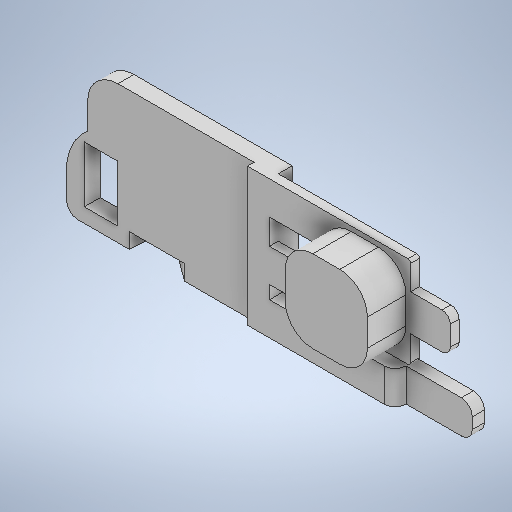
# Autodesk Inventor part: Botão Liga Desliga Monitor LG E2011
Saved by Autodesk Inventor 2025.3 (Build 293356000, 356)
## iProperties
Created: 2025-07-08
Part Number: Botão Liga Desliga Monitor LG E2011
Material: Genérico
Document SubType Name: Modeling
Designer: user
Density: 1 g/cm^3
Appearance: Padrão
Author: user
## iProperties of the stored document Botão Liga Desliga Monitor LG E2011_3DPrint.ipt
Created: 2025-07-08
Part Number: Botão Liga Desliga Monitor LG E2011_3DPrint
Material: Genérico
Document SubType Name: Modeling
Designer: user
Density: 1 g/cm^3
Appearance: Padrão
Author: user
Autodesk Inventor part; units mm, degrees
ref_plane "YZ Plane" through (0, 0, 0) normal (1, 0, 0) x (0, 1, 0)
ref_plane "XZ Plane" through (0, 0, 0) normal (0, 1, 0) x (-1, 0, 0)
ref_plane "XY Plane" through (0, 0, 0) normal (0, 0, 1) x (1, 0, 0)
sketch "Esboço1" plane through (0, 0, 0) normal (0, 0, 1) x (1, 0, 0)
  line L0 (0, 0) -> (36.4, 0)
  line L1 (0, 6.25) -> (36.4, 6.25)
  line L2 (36.4, 6.25) -> (36.4, -6.25)
  line L3 (36.4, -6.25) -> (0, -6.25)
  line L4 (0, -6.25) -> (0, 6.25)
  dimension "d0" = 36.4
  constraints: 10 end point, 2 horizontal, 2 parallel, 1 perpendicular
  measures "d0" distance of L0.start L0.end
extrude "Extrusão1" add sketch "Esboço1" along normal blind 2.65
sketch "Esboço2" plane through (0, 0, 2.65) normal (0, 0, 1) x (1, 0, 0)
  line L0 (0, -6.25) -> (36.4, -6.25) projected
  line L1 (19, -6.25) -> (19, -16.3254)
  line L2 (36.4, 6.25) -> (0, 6.25) projected
  line L3 (19, -6.25) -> (0, -6.25)
  line L4 (0, -6.25) -> (0, 6.25)
  line L5 (0, 6.25) -> (19, 6.25)
  line L6 (19, 6.25) -> (19, -6.25)
  line L7 (36.4, -6.25) -> (36.4, 6.25) projected
  line L8 (17, -6.25) -> (12.9263, -12.0226)
  line L9 (17, -6.25) -> (0, -6.25)
  line L10 (0, -6.25) -> (0, 6.25)
  line L11 (0, 6.25) -> (17, 6.25)
  line L12 (17, 6.25) -> (17, -6.25)
  point P0 (0, 0)
  dimension "d6" = 17.4
  constraints: 20 end point, 4 parallel, 2 horizontal, 2 perpendicular, 2 point on line
  measures "d6" distance between parallel lines of L7 L1
extrude "Extrusão2" cut sketch "Esboço2" against normal blind 0.6 contours L4 L2 L12 L0
sketch "Esboço3" plane through (0, 0, 2.05) normal (0, 0, 1) x (1, 0, 0)
  line L0 (17, 6.25) -> (17, -6.25) projected
  line L1 (17, 6.25) -> (1.9, 6.25)
  line L2 (36.4, 6.25) -> (0, 6.25) projected
  line L3 (1.9, 6.25) -> (1.9, 17.1493)
  line L4 (1.9, 6.25) -> (1.9, 0.15)
  line L5 (0, 6.25) -> (0, -6.25) projected
  line L6 (0, -6.25) -> (36.4, -6.25) projected
  line L7 (0, -4.95) -> (1.6, -4.95)
  line L8 (1.6, -4.95) -> (1.6, 0.15)
  line L9 (1.6, 0.15) -> (1.9, 0.15)
  line L10 (1.6, -4.95) -> (1.6, -7.116)
  line L11 (1.6, -4.95) -> (4.6, -4.95)
  line L12 (4.6, -4.95) -> (4.6, 0.15)
  line L13 (4.6, 0.15) -> (1.6, 0.15)
  line L14 (1.6, 0.15) -> (1.6, -4.95)
  line L15 (0, 0.15) -> (0, -2.35)
  line L16 (1.6, 0.15) -> (1.2464, 0.5036)
  line L17 (1.6, 0.15) -> (2.1, 0.15) construction
  line L18 (1.9, 0.15) -> (1.9, 1.15)
  arc A0 (1.9, 1.15) -> (0, -2.35) centre (5.3437, -2.9852) ccw
  point P0 (0, 0)
  dimension "d11" = 6.1
  dimension "d13" = 1.6
  dimension "d14" = 3
  dimension "d15" = 1.9
  dimension "d16" = 2.5
  dimension "d17" = 0.5
  dimension "d18" = 135
  dimension "d19" = 1
  constraints: 30 end point, 6 point on line, 3 horizontal, 3 perpendicular, 2 parallel, 2 point on circle, 2 vertical, 1 centre point, 1 equal length
  measures "d11" distance of L1.end L4.end
  measures "d13" distance of L7.start L7.end
  measures "d14" distance of L13.end L12.end
  measures "d15" distance between parallel lines of L5 L4
  measures "d16" distance of L15.start L15.end
  measures "d17" distance of L13.end L16.end
  measures "d18" angle of L17 L16
  measures "d19" distance of L4.end L18.end
extrude "Extrusão3" cut sketch "Esboço3" against normal blind 3 contours L4 A0 L5 L2 | L8 L9 L13 L12 L11
fillet "Arredondamento1" radius 2.75 1 edges at (1.9, 6.25, 1.025)
fillet "Arredondamento2" radius 1 1 edges at (0, -6.25, 1.025)
sketch "Esboço4" plane through (36.4, -6.25, 0) normal (0, -1, 0) x (1, 0, 0)
  line L0 (-30.7, 2.05) -> (-30.7, 6.0011)
  line L1 (-36.4, 0) -> (-30.6, 0)
  line L2 (-31.8, 0) -> (-34.8, 0) projected
  line L3 (-30.7, 2.05) -> (-30.6, 0)
  line L4 (-30.6, 0) -> (-27.55, 0)
  line L5 (0, 0) -> (-31.75, 0) projected
  line L6 (-27.55, 0) -> (-27.55, 0.7)
  line L7 (-30.7, 2.05) -> (-25.7, 2.05)
  line L8 (-31.75, 2.05) -> (-19.4, 2.05) projected
  line L9 (-27.55, 0.7) -> (-25.7, 2.05)
  point P0 (-36.4, 2.05)
  dimension "d25" = 5.8
  dimension "d26" = 3.05
  dimension "d27" = 0.7
  dimension "d28" = 5
  constraints: 14 end point, 2 point on line, 1 collinear, 1 vertical
  measures "d25" distance of L1.start L1.end
  measures "d26" distance of L1.end L4.end
  measures "d27" distance of L4.end L6.end
  measures "d28" distance of L0.start L7.end
extrude "Extrusão4" cut sketch "Esboço4" against normal blind 1.4
sketch "Esboço5" plane through (0, 0, 0) normal (0, 0, -1) x (-1, 0, 0)
  line L0 (-17, -6.25) -> (-10.7, -6.25) projected
  line L1 (-17, 1.25) -> (-6.1, 1.25)
  line L2 (-4.6, -4.95) -> (-4.6, 0.15) projected
  line L3 (-4.6, -0.25) -> (-4.6, -6.25)
  line L4 (-17, 6.25) -> (-4.6, 6.25)
  arc A0 (-1.9, 3.5) -> (-4.65, 6.25) centre (-4.65, 3.5) ccw projected
  arc A1 (-4.6, 6.2495) -> (-4.65, 6.25) centre (-4.65, 3.5) ccw
  line L5 (-1.9, 1.15) -> (-1.9, 3.5) projected
  line L6 (-1.9, 3.5) -> (-1.9, 1.15)
  arc A2 (0, -2.35) -> (-1.9, 1.15) centre (-5.3437, -2.9852) ccw projected
  line L7 (0, -2.35) -> (0, -5.25) projected
  line L8 (0, -2.35) -> (0, -5.25)
  line L9 (-1, -6.25) -> (-5.8, -6.25) projected
  line L10 (-1, -6.25) -> (-4.6, -6.25)
  arc A3 (-1, -6.25) -> (0, -5.25) centre (-1, -5.25) ccw projected
  arc A4 (-1, -6.25) -> (0, -5.25) centre (-1, -5.25) ccw
  arc A5 (0, -3.6203) -> (-1.9, 1.15) centre (-5.3437, -2.9852) ccw
  line L11 (-6.1, 1.25) -> (-6.1, -0.25)
  arc A6 (-4.6, -0.25) -> (-6.1, 1.25) centre (-6.1, -0.25) ccw
  line L12 (-17, -6.25) -> (-19, -6.25)
  line L13 (-17, -6.25) -> (-36.4, -6.25) projected
  line L14 (-19, -6.25) -> (-19, 6.25)
  line L15 (-19, 6.25) -> (-17, 6.25)
  line L16 (-17, 1.25) -> (-19, 1.25)
  point P0 (0, 0)
  point P1 (-4.6, -0.25)
  dimension "d31" = 7.5
  dimension "d36" = 2
  constraints: 22 end point, 8 point on circle, 6 point on line, 5 perpendicular, 4 centre point, 4 coincident, 3 collinear, 1 horizontal
  measures "d31" distance of L0.start L1.start
  measures "d36" distance of L0.start L12.end
extrude "Extrusão5" cut sketch "Esboço5" against normal blind 0.6 contours L16 L14 L15 L4 A0 L5 A2 L7 A3 L9 L3 L2 A6 L1
sketch "Esboço6" plane through (0, 0, 2.65) normal (0, 0, 1) x (1, 0, 0)
  line L0 (17, -6.25) -> (36.4, -6.25) projected
  line L1 (36.4, -6.25) -> (18.95, -6.25)
  line L2 (18.95, -6.25) -> (18.95, -3.25)
  line L3 (18.95, -3.25) -> (36.4, -3.25)
  line L4 (36.4, -3.25) -> (36.4, -6.25)
  line L5 (36.4, -3.25) -> (30.4, -3.25)
  line L6 (30.4, -3.25) -> (30.4, -6.25)
  line L7 (30.4, -6.25) -> (36.4, -6.25)
  line L8 (36.4, -6.25) -> (36.4, -3.25)
  point P0 (0, 0)
  dimension "d37" = 17.45
  dimension "d38" = 3
  dimension "d39" = 6
  constraints: 16 end point, 4 parallel, 2 horizontal, 2 perpendicular, 1 point on line
  measures "d37" distance of L2.end L3.end
  measures "d38" distance of L1.end L2.end
  measures "d39" distance of L7.end L6.end
extrude "Extrusão6" cut sketch "Esboço6" against normal blind 1 contours L6 L3 L4 L0
sketch "Esboço7" plane through (0, 0, 0) normal (0, 0, -1) x (-1, 0, 0)
  line L0 (-8.85, -6.25) -> (-36.4, -6.25) projected
  line L1 (-36.4, -6.25) -> (-29.3, -6.25)
  line L2 (-29.3, -6.25) -> (-29.3, -3.25)
  line L3 (-29.3, -3.25) -> (-36.4, -3.25)
  line L4 (-36.4, -3.25) -> (-36.4, -6.25)
  point P0 (0, 0)
  dimension "d42" = 7.1
  constraints: 8 end point, 2 parallel, 1 horizontal, 1 perpendicular
  measures "d42" distance of L3.end L2.end
extrude "Extrusão7" cut sketch "Esboço7" against normal blind 0.55
fillet "Arredondamento3" radius 1 1 edges at (30.4, -4.75, 2.65)
fillet "Arredondamento4" radius 2.5 1 edges at (29.3, -4.75, 0)
sketch "Esboço8" plane through (0, 0, 2.65) normal (0, 0, 1) x (1, 0, 0)
  line L0 (19, 6.25) -> (31.8, 6.25)
  line L1 (31.8, -2.05) -> (19, -2.05)
  line L2 (31.8, 3.775) -> (36.4, 3.775)
  line L3 (36.4, 0.475) -> (31.8, 0.475)
  line L4 (31.8, 6.25) -> (31.8, 3.775)
  line L5 (31.8, 0.475) -> (31.8, -2.05)
  line L6 (31.8, 6.25) -> (31.8, 3.775)
  line L7 (31.8, 0.475) -> (31.8, -2.05)
  line L8 (19, 6.25) -> (19, -2.05)
  line L9 (36.4, -3.25) -> (36.4, 6.25) projected
  line L10 (36.4, -3.25) -> (29.3, -3.25) projected
  line L11 (36.4, -3.25) -> (19, -3.25)
  line L12 (19, -3.25) -> (19, -2.05)
  line L13 (36.4, -3.25) -> (36.4, 0.475)
  line L14 (36.4, 3.775) -> (36.4, 6.25)
  line L15 (36.4, 3.775) -> (36.4, 0.475)
  line L16 (36.4, -3.25) -> (36.4, 6.25) projected
  line L17 (31.8, 3.775) -> (36.4, 3.775)
  line L18 (36.4, 3.775) -> (36.4, 6.25)
  line L19 (36.4, 6.25) -> (31.8, 6.25)
  line L20 (31.8, 6.25) -> (31.8, 3.775)
  point P0 (0, 0)
  dimension "d51" = 8.3
  dimension "d54" = 17.4
  constraints: 36 end point, 4 point on line, 3 horizontal, 3 parallel, 2 collinear, 2 perpendicular, 2 vertical
  measures "d51" distance of L5.end L4.start
  measures "d54" distance between parallel lines of L9 L8
extrude "Extrusão8" cut sketch "Esboço8" against normal blind 3 contours L19 L9 L2 L4 | L1 L5 L3 L9 L10 L11 L12
fillet "Arredondamento5" radius 0.75 2 edges at (36.4, 0.475, 1.325) (36.4, 3.775, 1.325)
fillet "Arredondamento6" radius 1 2 edges at (36.4, -6.25, 1.1) (36.4, -3.25, 1.1)
sketch "Esboço9" plane through (0, 0, 2.65) normal (0, 0, 1) x (1, 0, 0)
  line L0 (19, 6.25) -> (19, 3.25)
  line L1 (31.8, -2.05) -> (19, -2.05) projected
  line L2 (19, -2.05) -> (19, 0.95)
  line L3 (19, 3.25) -> (23.5, 3.25)
  line L4 (23.5, 3.25) -> (23.5, 0.95)
  line L5 (23.5, 0.95) -> (19, 0.95)
  line L6 (19, 0.95) -> (19, 3.25)
  line L7 (23.5, 2.1) -> (23.5, 6.25)
  line L8 (23.5, 6.25) -> (31.8, 6.25)
  line L9 (31.8, 6.25) -> (31.8, -2.05)
  line L10 (31.8, -2.05) -> (23.5, -2.05)
  line L11 (23.5, -2.05) -> (23.5, 6.25)
  line L12 (23.725, 6.025) -> (31.575, 6.025)
  line L13 (31.575, 6.025) -> (31.575, -1.825)
  line L14 (31.575, -1.825) -> (23.725, -1.825)
  line L15 (23.725, -1.825) -> (23.725, 6.025)
  point P0 (0, 0)
  dimension "d59" = 3
  dimension "d60" = 3
  dimension "d63" = 8.3
  dimension "d66" = 7.85
  dimension "d67" = 7.85
  dimension "d70" = 4.5
  dimension "d71" = 0.225
  constraints: 30 end point, 6 parallel, 3 horizontal, 3 perpendicular, 1 midpoint, 1 point on line, 1 vertical
  measures "d59" distance of L0.start L0.end
  measures "d60" distance of L1.end L2.end
  measures "d63" distance of L9.end L10.end
  measures "d66" distance of L13.end L14.end
  measures "d67" distance of L12.end L13.end
  measures "d70" distance between parallel lines of L4 L6
  measures "d71" distance between parallel lines of L9 L13
extrude "Extrusão9" cut sketch "Esboço9" against normal blind 3 contours L5 L6 L3 L4
sketch "Esboço10" plane through (0, 0, 0) normal (0, 0, -1) x (-1, 0, 0)
  line L0 (-19, -2.05) -> (-19, -3.25) projected
  line L1 (-19, -2.05) -> (-23.5, -2.05)
  line L2 (-23.5, 0.95) -> (-19, 0.95)
  line L3 (-19, 0.95) -> (-19, -2.05)
  line L4 (-23.5, 3.25) -> (-19, 3.25) projected
  line L5 (-31.8, 6.25) -> (-19, 6.25) projected
  line L6 (-19, 3.25) -> (-23.5, 3.25)
  line L7 (-23.5, 6.25) -> (-19, 6.25)
  line L8 (-19, 6.25) -> (-19, 3.25)
  line L9 (-31.8, -2.05) -> (-31.8, 0.475) projected
  line L10 (-35.65, 3.775) -> (-31.8, 3.775) projected
  line L11 (-31.8, 0.475) -> (-35.65, 0.475)
  line L12 (-35.65, 3.775) -> (-31.8, 3.775)
  arc A0 (-35.65, 3.775) -> (-36.4, 3.025) centre (-35.65, 3.025) ccw projected
  arc A1 (-35.65, 3.775) -> (-36.3655, 3.25) centre (-35.65, 3.025) ccw
  arc A2 (-36.4, 1.225) -> (-35.65, 0.475) centre (-35.65, 1.225) ccw projected
  line L13 (-31.8, 3.775) -> (-31.8, 6.25) projected
  line L14 (-23.5, -2.05) -> (-31.8, -2.05)
  line L15 (-31.8, 6.25) -> (-23.5, 6.25)
  line L16 (-23.5, 3.25) -> (-23.5, 0.95)
  line L17 (-31.8, -2.05) -> (-31.8, 0.475)
  line L18 (-31.8, 3.775) -> (-31.8, 6.25)
  line L19 (-36.4, 1.225) -> (-36.4, 3.025) projected
  line L20 (-36.4, 1.225) -> (-36.4, 3.025)
  point P0 (0, 0)
  constraints: 28 end point, 6 parallel, 4 horizontal, 4 point on line, 2 perpendicular, 2 point on circle, 1 centre point, 1 coincident, 1 collinear
extrude "Extrusão10" cut sketch "Esboço10" against normal blind 1.85
sketch "Esboço11" plane through (0, 0, 2.65) normal (0, 0, 1) x (1, 0, 0)
  line L0 (31.8, 6.25) -> (19, 6.25)
  line L1 (23.5, 3.25) -> (23.5, 0.95)
  line L2 (19, 6.25) -> (23.5, 6.25)
  line L3 (23.5, 6.25) -> (23.5, 3.25)
  line L4 (23.5, 3.25) -> (19, 3.25)
  line L5 (19, 3.25) -> (19, 6.25)
  line L6 (31.8, -2.05) -> (31.8, 0.475)
  line L7 (23.5, 6.25) -> (31.8, 6.25)
  line L8 (31.8, 6.25) -> (31.8, -2.05)
  line L9 (31.8, -2.05) -> (23.5, -2.05)
  line L10 (23.5, -2.05) -> (23.5, 6.25)
  line L11 (23.925, 5.825) -> (31.375, 5.825)
  line L12 (31.375, 5.825) -> (31.375, -1.625)
  line L13 (31.375, -1.625) -> (23.925, -1.625)
  line L14 (23.925, -1.625) -> (23.925, 5.825)
  point P0 (0, 0)
  dimension "d96" = 0.425
  dimension "d97" = 0.425
  dimension "d98" = 0.425
  dimension "d99" = 0.425
  constraints: 30 end point, 2 parallel, 1 horizontal, 1 perpendicular, 1 vertical
  measures "d96" distance between parallel lines of L0 L11
  measures "d97" distance between parallel lines of L9 L13
  measures "d98" distance between parallel lines of L1 L14
  measures "d99" distance between parallel lines of L8 L12
fillet "Arredondamento7" radius 0.25 1 edges at (31.8, -2.05, 2.25)
fillet "Arredondamento8" radius 0.25 1 edges at (31.8, 6.25, 2.25)
sketch "Esboço12" plane through (0, 0, 2.65) normal (0, 0, 1) x (1, 0, 0)
  line L0 (36.4, 3.775) -> (35.4, 3.775)
  line L1 (35.4, 3.775) -> (35.4, 0.475)
  line L2 (31.8, 0.475) -> (35.65, 0.475) projected
  line L3 (35.4, 0.475) -> (36.4, 0.475)
  line L4 (36.4, 0.475) -> (36.4, 3.775)
  point P0 (0, 0)
  dimension "d89" = 1
  constraints: 8 end point, 2 horizontal, 2 perpendicular, 1 point on line
  measures "d89" distance of L0.start L0.end
extrude "Extrusão12" cut sketch "Esboço12" against normal blind 3
fillet "Arredondamento10" radius 0.75 2 edges at (35.4, 3.775, 2.25) (35.4, 0.475, 2.25)
extrude "Extrusão13" add sketch "Esboço11" along normal blind 3.5 contours L11 L12 L13 L14
fillet "Arredondamento11" radius 2.5 4 edges at (23.925, 5.825, 4.4) (23.925, -1.625, 4.4) (31.375, -1.625, 4.4) (31.375, 5.825, 4.4)
